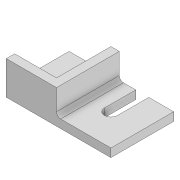
# Autodesk Inventor part: Laptop-ecke
Saved by Autodesk Inventor 2022 (Build 260153000, 153)
## iProperties
Created: 2024-04-12
Part Number: Laptop-ecke
Material: Generic
Document SubType Name: Modeling
Designer: LaptopJR
Density: 1 g/cm^3
Appearance: Default
Author: LaptopJR
## iProperties of the stored document Laptop-ecke_3DPrint.ipt
Created: 2024-04-12
Part Number: Laptop-ecke_3DPrint
Material: Generic
Document SubType Name: Modeling
Designer: LaptopJR
Density: 1 g/cm^3
Appearance: Default
Author: LaptopJR
Autodesk Inventor part; units mm, degrees
ref_plane "YZ Plane" through (0, 0, 0) normal (1, 0, 0) x (0, 1, 0)
ref_plane "XZ Plane" through (0, 0, 0) normal (0, 1, 0) x (-1, 0, 0)
ref_plane "XY Plane" through (0, 0, 0) normal (0, 0, 1) x (1, 0, 0)
sketch "Sketch1" plane through (0, 0, 0) normal (0, 1, 0) x (-1, 0, 0)
  line L0 (0, 0) -> (-50, 0)
  line L1 (-50, 0) -> (-50, -30)
  line L2 (0, -30) -> (0, 0)
  line L3 (-50, -15) -> (-35, -15) construction
  arc A0 (-31.9, -15) -> (-38.1, -15) centre (-35, -15) ccw
  line L4 (-31.9, -15) -> (-31.9, -30)
  line L5 (-38.1, -15) -> (-38.1, -30)
  line L6 (-50, -30) -> (-38.1, -30)
  line L7 (-31.9, -30) -> (0, -30)
  dimension "d0" = 15
  dimension "d1" = 6.2
  dimension "d2" = 30
  dimension "d3" = 50
  constraints: 16 end point, 5 perpendicular, 3 parallel, 2 horizontal, 2 point on circle, 1 centre point, 1 coincident, 1 midpoint, 1 point on line, 1 tangent
  measures "d0" distance of L3.start L3.end
  measures "d1" diameter of A0
  measures "d2" distance of L0.end L1.end
  measures "d3" distance of L0.start L0.end
extrude "Extrusion1" add sketch "Sketch1" along normal blind 4
sketch "Sketch2" plane through (0, 4, 0) normal (0, 1, 0) x (1, 0, 0)
  line L0 (31.9, 30) -> (0, 30) projected
  line L1 (20, 30) -> (20, 4)
  line L2 (20, 4) -> (0, 4)
  line L3 (0, 30) -> (0, 0) projected
  line L4 (50, 0) -> (50, 30) projected
  line L5 (0, 0) -> (50, 0) projected
  line L6 (24, 30) -> (24, 0)
  dimension "d6" = 30
  dimension "d7" = 4
  dimension "d8" = 4
  constraints: 6 end point, 4 point on line, 2 perpendicular, 1 vertical
  measures "d6" distance between parallel lines of L4 L1
  measures "d7" distance between parallel lines of L5 L2
  measures "d8" distance between parallel lines of L6 L1
extrude "Extrusion2" add sketch "Sketch2" along normal blind 12 contours L6 L5 L3 L2 L1 L0
fillet "Fillet1" radius 2 3 edges at (20, 4, -17) (10, 4, -4) (24, 4, -15)
body "Solid1"
